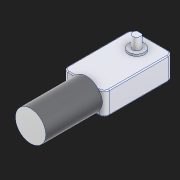
# Autodesk Inventor part: TSINY TS-42GZ495
Saved by Autodesk Inventor 2017 (Build 210142000, 142)
## iProperties
Created: 2018-04-11
Part Number: TSINY TS-42GZ495
Material: Generic
Document SubType Name: Modeling
Designer: Zach
Density: 1 g/cm^3
Appearance: Aluminum - Flat
Author: Zach
Autodesk Inventor part; units mm, degrees
ref_plane "YZ Plane" through (0, 0, 0) normal (1, 0, 0) x (0, 1, 0)
ref_plane "XZ Plane" through (0, 0, 0) normal (0, 1, 0) x (-1, 0, 0)
ref_plane "XY Plane" through (0, 0, 0) normal (0, 0, 1) x (1, 0, 0)
sketch "Sketch1" plane through (0, 0, 0) normal (0, 0, 1) x (1, 0, 0)
  circle A0 centre (0, 0) radius 15.5
  dimension "d0" = 31
  constraints: 1 centre point, 1 coincident
  measures "d0" diameter of A0
extrude "Extrusion1" add sketch "Sketch1" along normal blind 57.1
sketch "Sketch2" plane through (0, 0, 0) normal (0, 1, 0) x (-1, 0, 0)
  line L0 (24, -70) -> (-18, -70)
  line L1 (-18, -70) -> (-18, 0)
  line L2 (-18, 0) -> (24, 0)
  line L3 (24, 0) -> (24, -70)
  line L4 (3, 0) -> (3, -70) construction
  point P0 (0, 0)
  dimension "d3" = 70
  dimension "d4" = 42
  dimension "d5" = 3
  constraints: 10 end point, 2 midpoint, 2 parallel, 1 horizontal, 1 perpendicular, 1 point on line
  measures "d3" distance of L0.end L1.end
  measures "d4" distance of L1.end L2.end
  measures "d5" distance from line of point (0, 0) L4
extrude "Extrusion2" add sketch "Sketch2" against normal blind 13 and the other way blind 10
sketch "Sketch3" plane through (0, -13, 0) normal (0, -1, 0) x (1, 0, 0)
  line L0 (-24, -70) -> (18, -70) construction
  line L1 (18, -70) -> (18, 0) construction
  line L2 (18, 0) -> (8.441, 0) construction
  line L3 (-8.441, 0) -> (8.441, 0) construction
  line L4 (-8.441, 0) -> (-24, 0) construction
  line L5 (-24, 0) -> (-24, -70) construction
  line L6 (18, -70) -> (-24, -70) construction
  line L7 (-3, -70) -> (-3, 0) construction
  line L8 (-11.8427, 0) -> (11.8427, 0) construction
  circle A0 centre (-3, -54) radius 4
  line L9 (6, -62) -> (-12, -62) construction
  line L10 (-12, -62) -> (-12, -29) construction
  line L11 (-12, -29) -> (6, -29) construction
  line L12 (6, -29) -> (6, -62) construction
  circle A1 centre (6, -62) radius 1.5
  circle A2 centre (-12, -62) radius 1.5
  circle A3 centre (-12, -29) radius 1.5
  circle A4 centre (6, -29) radius 1.5
  point P0 (0, 0)
  point P1 (-3, -62)
  dimension "d10" = 8
  dimension "d11" = 33
  dimension "d12" = 18
  dimension "d13" = 8
  dimension "d14" = 8
  dimension "d15" = 3
  dimension "d16" = 3
  dimension "d17" = 3
  dimension "d18" = 3
  constraints: 10 end point, 5 centre point, 4 coincident, 2 midpoint, 2 parallel, 2 perpendicular, 2 point on line, 1 horizontal, 1 vertical alignment
  measures "d10" diameter of A0
  measures "d11" distance of L9.end L10.end
  measures "d12" distance of L9.start L9.end
  measures "d13" distance from line of L9 A0.centre
  measures "d14" distance between parallel lines of L0 L9
  measures "d15" diameter of A1
  measures "d16" diameter of A2
  measures "d17" diameter of A3
  measures "d18" diameter of A4
extrude "Extrusion3" cut sketch "Sketch3" against normal blind 15
sketch "Sketch4" plane through (0, -13, 0) normal (0, -1, 0) x (1, 0, 0)
  circle A0 centre (-3, -54) radius 4 projected
  point P0 (0, 0)
extrude "Extrusion4" add sketch "Sketch4" along normal blind 14 and the other way blind 15
sketch "Sketch5" plane through (-3, -27, -54) normal (0, -1, 0) x (1, 0, 0)
  circle A0 centre (0, 0) radius 4 construction
  line L0 (2.6458, -3) -> (-2.6458, -3)
  arc A1 (-2.6458, -3) -> (2.6458, -3) centre (0, 0) ccw
  point P0 (3, 54)
  dimension "d25" = 3
  constraints: 4 point on circle, 2 end point, 1 centre point, 1 concentric, 1 horizontal
  measures "d25" distance from line of L0 A0.centre
extrude "Extrusion5" cut sketch "Sketch5" against normal blind 8
sketch "Sketch6" plane through (0, -13, 0) normal (0, -1, 0) x (1, 0, 0)
  arc A0 (-0.3542, -57) -> (-5.6458, -57) centre (-3, -54) ccw projected
  circle A1 centre (-3, -54) radius 8
  circle A2 centre (6, -62) radius 1.5 projected
  circle A3 centre (-12, -62) radius 1.5 projected
  circle A4 centre (-12, -29) radius 1.5 projected
  circle A5 centre (6, -29) radius 1.5 projected
  circle A6 centre (6, -62) radius 4.5
  circle A7 centre (-12, -62) radius 1.5 projected
  circle A8 centre (-12, -62) radius 4.5
  circle A9 centre (-12, -29) radius 4
  circle A10 centre (6, -29) radius 4
  point P0 (0, 0)
  dimension "d28" = 16
  dimension "d31" = 9
  dimension "d32" = 9
  dimension "d33" = 8
  dimension "d34" = 8
  constraints: 5 centre point, 5 coincident
  measures "d28" diameter of A1
  measures "d31" diameter of A6
  measures "d32" diameter of A8
  measures "d33" diameter of A9
  measures "d34" diameter of A10
extrude "Extrusion6" add sketch "Sketch6" along normal blind 2
fillet "Fillet1" radius 5 4 edges at (18, -1.5, -70) (18, -1.5, 0) (-24, -1.5, -70) (-24, -1.5, 0)
fillet "Fillet2" radius 1 18 edges at (16.5355, -13, -68.5355) (18, -13, -35) (16.5355, -13, -1.4645) (-13.7205, -13, 0) (10.7205, -13, 0) (-22.5355, -13, -68.5355) (-24, -13, -35) (-22.5355, -13, -1.4645) (-3, -13, -70) (-22.5355, 10, -68.5355) (-24, 10, -35) (-22.5355, 10, -1.4645) (12.4214, 10, 0) (-15.4214, 10, 0) (16.5355, 10, -68.5355) (18, 10, -35) (16.5355, 10, -1.4645) (-3, 10, -70)
sketch "Sketch7" plane through (0, 10, 0) normal (0, 1, 0) x (1, 0, 0)
  circle A0 centre (-3, 54) radius 4 projected
  arc A1 (-5.6458, 57) -> (-0.3542, 57) centre (-3, 54) ccw projected
  arc A2 (-0.3542, 57) -> (-5.6458, 57) centre (-3, 54) ccw projected
  point P0 (0, 0)
extrude "Extrusion7" add sketch "Sketch7" along normal blind 14
sketch "Sketch8" plane through (0, 10, 0) normal (0, 1, 0) x (1, 0, 0)
  circle A0 centre (-3, 54) radius 4 projected
  circle A1 centre (-3, 54) radius 8
  point P0 (0, 0)
  dimension "d39" = 16
  constraints: 1 centre point, 1 coincident
  measures "d39" diameter of A1
extrude "Extrusion8" add sketch "Sketch8" along normal blind 2
sketch "Sketch9" plane through (-3, 24, -54) normal (0, 1, 0) x (1, 0, 0)
  line L0 (-2.6458, 3) -> (2.6458, 3) projected
  arc A0 (2.6458, 3) -> (-2.6458, 3) centre (0, 0) ccw projected
  point P0 (3, -54)
extrude "Extrusion9" cut sketch "Sketch9" against normal blind 8
sketch "Sketch11" plane through (-3, -19, -54) normal (0, -1, 0) x (1, 0, 0)
  circle A0 centre (0, 0) radius 4 projected
  point P0 (3, 54)
extrude "Extrusion11" add sketch "Sketch11" along normal blind 8
sketch "Sketch15" plane through (-3, -27, -54) normal (0, -1, 0) x (1, 0, 0)
  circle A0 centre (0, 0) radius 4 projected
  line L0 (2.6458, -3) -> (-2.6458, -3) projected
  point P0 (3, 54)
extrude "Extrusion15" cut sketch "Sketch15" against normal blind 8 contours L0 A0 picked at (-0.6179, -3.1815)
body "Solid1"
